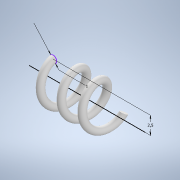
# Autodesk Inventor part: Пружина
Saved by Autodesk Inventor 2022 (Build 260153000, 153)
## iProperties
Created: 2021-04-26
Part Number: Пружина
Material: Типовые
Document SubType Name: Modeling
Designer: lbfas
Density: 1 g/cm^3
Appearance: По умолчанию
Author: lbfas
Autodesk Inventor part; units mm, degrees
ref_plane "YZ Plane" through (0, 0, 0) normal (1, 0, 0) x (0, 1, 0)
ref_plane "XZ Plane" through (0, 0, 0) normal (0, 1, 0) x (-1, 0, 0)
ref_plane "XY Plane" through (0, 0, 0) normal (0, 0, 1) x (1, 0, 0)
sketch "Эскиз1" plane through (0, 0, 0) normal (0, 0, 1) x (1, 0, 0)
  circle A0 centre (-13.2216, 1.6848) radius 0.5
  line L0 (-4.6945, -0.0652) -> (-13.7216, -0.0652)
  dimension "d0" = 1
  dimension "d1" = 1.75
  constraints: 2 end point, 1 centre point, 1 horizontal
  measures "d0" diameter of A0
  measures "d1" distance from line of L0 A0.centre
coil "Пружина1" sketch "Эскиз1" operation add axis through (-4.6945, -0.0652, 0) along (1, 0, 0) pitch 3 turns 2.666667 hand right
